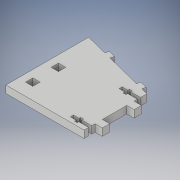
# Autodesk Inventor part: pinball-case-left-wal-scaledl
Saved by Autodesk Inventor 2017 (Build 210142000, 142)
## iProperties
Created: 2017-02-27
Part Number: pinball-case-left-wal-scaledl
Material: Generic
Document SubType Name: Modeling
Designer: John
Density: 1 g/cm^3
Appearance: Default
Author: John
Autodesk Inventor part; units mm, degrees
ref_plane "YZ Plane" through (0, 0, 0) normal (1, 0, 0) x (0, 1, 0)
ref_plane "XZ Plane" through (0, 0, 0) normal (0, 1, 0) x (-1, 0, 0)
ref_plane "XY Plane" through (0, 0, 0) normal (0, 0, 1) x (1, 0, 0)
sketch "Sketch1" plane through (0, 0, 0) normal (0, 1, 0) x (-1, 0, 0)
  line L0 (0, 0) -> (-70, 0)
  line L1 (-70, 0) -> (-70, -50)
  line L2 (-70, -50) -> (0, -50)
  line L3 (0, -50) -> (0, 0)
  line L4 (0, -50) -> (0, -67.7966)
  line L5 (0, -67.7966) -> (-70, -50)
  dimension "d0" = 70
  dimension "d1" = 50
  dimension "d45" = 14.264
  constraints: 12 end point, 2 parallel, 1 horizontal, 1 perpendicular, 1 vertical
  measures "d0" distance of L2.end L1.end
  measures "d1" distance of L1.end L0.end
  measures "d45" angle of L2 L5
extrude "Extrusion1" add sketch "Sketch1" along normal blind 6
sketch "Sketch2" plane through (0, 6, 0) normal (0, 1, 0) x (1, 0, 0)
  line L0 (70, 50) -> (58.37, 52.9568) construction
  line L1 (70, 50) -> (0, 67.7966) construction
  line L2 (58.37, 52.9568) -> (52.555, 54.4352)
  line L3 (52.555, 54.4352) -> (53.2942, 57.3427)
  line L4 (53.2942, 57.3427) -> (59.1092, 55.8643)
  line L5 (59.1092, 55.8643) -> (58.37, 52.9568)
  line L6 (23.4799, 61.8271) -> (17.6649, 63.3055)
  line L7 (17.6649, 63.3055) -> (18.4041, 66.213)
  line L8 (18.4041, 66.213) -> (24.2191, 64.7346)
  line L9 (24.2191, 64.7346) -> (23.4799, 61.8271)
  point P0 (0, 0)
  dimension "d9" = 12
  dimension "d10" = 6
  dimension "d11" = 3
  dimension "d15" = 6
  dimension "d16" = 3
  dimension "d17" = 30
  constraints: 18 end point, 4 parallel, 3 point on line, 2 perpendicular
  measures "d9" distance of L0.start L0.end
  measures "d10" distance of L0.end L2.end
  measures "d11" distance of L2.end L3.end
  measures "d15" distance of L6.start L6.end
  measures "d16" distance of L6.end L7.end
  measures "d17" distance between parallel lines of L9 L3
extrude "Extrusion2" add sketch "Sketch2" against normal blind 6
sketch "Sketch3" plane through (0, 6, 0) normal (0, 1, 0) x (1, 0, 0)
  line L0 (70, 0) -> (70, 50) projected
  line L1 (70, 54) -> (64, 54)
  line L2 (64, 54) -> (64, 41)
  line L3 (64, 41) -> (70, 41)
  line L4 (70, 41) -> (70, 54)
  line L5 (70, 0) -> (64, 0)
  line L6 (64, 0) -> (64, 9)
  line L7 (64, 9) -> (70, 9)
  line L8 (70, 9) -> (70, 0)
  line L9 (70, 35) -> (64, 35)
  line L10 (64, 35) -> (64, 15)
  line L11 (64, 15) -> (70, 15)
  line L12 (70, 15) -> (70, 35)
  point P0 (0, 0)
  dimension "d18" = 6
  dimension "d20" = 6
  dimension "d21" = 9
  dimension "d22" = 6
  dimension "d23" = 6
  dimension "d27" = 20
  dimension "d36" = 13
  constraints: 24 end point, 6 parallel, 3 horizontal, 3 perpendicular, 1 point on line
  measures "d18" distance of L3.end L2.end
  measures "d20" distance of L6.end L7.end
  measures "d21" distance of L5.end L6.end
  measures "d22" distance between parallel lines of L3 L9
  measures "d23" distance between parallel lines of L7 L11
  measures "d27" distance of L9.end L10.end
  measures "d36" distance of L1.end L2.end
extrude "Extrusion3" cut sketch "Sketch3" along normal through all both and the other way through all
sketch "Sketch4" plane through (0, 6, 0) normal (0, 1, 0) x (1, 0, 0)
  line L0 (64, 0) -> (64, 9) projected
  line L1 (64, 6.25) -> (56, 6.25)
  line L2 (49, 6.25) -> (49, 3.75)
  line L3 (49, 3.75) -> (53.7, 3.75)
  line L4 (64, 3.75) -> (64, 6.25)
  line L5 (64, 9) -> (70, 9) projected
  line L6 (64, 43.75) -> (56, 43.75)
  line L7 (49, 43.75) -> (49, 46.25)
  line L8 (49, 46.25) -> (53.7, 46.25)
  line L9 (64, 46.25) -> (64, 43.75)
  line L10 (70, 41) -> (64, 41) projected
  line L11 (64, 41) -> (64, 51.5254) projected
  line L12 (56, 47.6) -> (53.7, 47.6)
  line L13 (53.7, 47.6) -> (53.7, 46.25)
  line L14 (53.7, 42.4) -> (56, 42.4)
  line L15 (56, 42.4) -> (56, 43.75)
  line L16 (53.7, 7.6) -> (56, 7.6)
  line L17 (56, 7.6) -> (56, 6.25)
  line L18 (56, 2.4) -> (53.7, 2.4)
  line L19 (53.7, 2.4) -> (53.7, 3.75)
  line L20 (53.7, 6.25) -> (53.7, 7.6)
  line L21 (53.7, 3.75) -> (53.7, 6.25) construction
  line L22 (56, 6.25) -> (56, 3.75) construction
  line L23 (56, 3.75) -> (56, 2.4)
  line L24 (56, 3.75) -> (64, 3.75)
  line L25 (53.7, 3.75) -> (56, 3.75) construction
  line L26 (56, 6.25) -> (53.7, 6.25) construction
  line L27 (53.7, 6.25) -> (49, 6.25)
  line L28 (53.7, 43.75) -> (53.7, 42.4)
  line L29 (53.7, 46.25) -> (53.7, 43.75) construction
  line L30 (53.7, 43.75) -> (49, 43.75)
  line L31 (56, 43.75) -> (53.7, 43.75) construction
  line L32 (56, 46.25) -> (56, 47.6)
  line L33 (56, 43.75) -> (56, 46.25) construction
  line L34 (53.7, 46.25) -> (56, 46.25) construction
  line L35 (56, 46.25) -> (64, 46.25)
  line L36 (6, 10) -> (12, 10)
  line L37 (12, 10) -> (12, 16)
  line L38 (12, 16) -> (6, 16)
  line L39 (6, 16) -> (6, 10)
  line L40 (6, 31) -> (12, 31)
  line L41 (12, 31) -> (12, 37)
  line L42 (12, 37) -> (6, 37)
  line L43 (6, 37) -> (6, 31)
  line L44 (0, 0) -> (64, 0) projected
  line L45 (0, 67.7966) -> (0, 0) projected
  point P0 (64, 45)
  dimension "d37" = 15
  dimension "d38" = 2.5
  dimension "d42" = 15
  dimension "d43" = 2.5
  dimension "d44" = 2.75
  dimension "d46" = 2.75
  dimension "d47" = 5.2
  dimension "d48" = 2.3
  dimension "d49" = 5.2
  dimension "d50" = 8
  dimension "d51" = 8
  dimension "d52" = 6
  dimension "d53" = 6
  dimension "d54" = 6
  dimension "d55" = 6
  dimension "d56" = 10
  dimension "d57" = 6
  dimension "d58" = 15
  constraints: 80 end point, 44 parallel, 14 perpendicular, 10 horizontal, 5 point on line, 3 equal length, 1 midpoint
  measures "d37" distance of L4.start L2.end
  measures "d38" distance of L2.end L2.start
  measures "d42" distance of L7.end L9.start
  measures "d43" distance of L7.start L7.end
  measures "d44" distance between parallel lines of L6 L10
  measures "d46" distance between parallel lines of L5 L1
  measures "d47" distance of L18.end L16.start
  measures "d48" distance of L16.start L16.end
  measures "d49" distance between parallel lines of L14 L12
  measures "d50" distance between parallel lines of L11 L32
  measures "d51" distance between parallel lines of L0 L17
  measures "d52" distance of L38.end L37.end
  measures "d53" distance of L37.end L36.end
  measures "d54" distance of L42.end L41.end
  measures "d55" distance of L41.end L40.end
  measures "d56" distance between parallel lines of L44 L36
  measures "d57" distance between parallel lines of L45 L39
  measures "d58" distance between parallel lines of L40 L38
extrude "Extrusion4" cut sketch "Sketch4" along normal through all both and the other way through all
equation "\"d15\" = d10"
equation "\"d16\" = d11"
equation "\"d18\" = d20"
equation "\"d42\" = d37"
equation "\"d43\" = d38"
equation "\"d44\" = d46"
equation "\"d50\" = d51"
equation "\"d54\" = d52"
body "Solid1"
